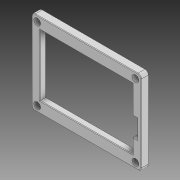
# Autodesk Inventor part: MainLid
Saved by Autodesk Inventor 2020 (Build 240168000, 168)
## iProperties
Created: 2021-01-12
Part Number: MainLid
Material: Generic
Document SubType Name: Modeling
Designer: DDeGo
Density: 1 g/cm^3
Appearance: Default
Author: DDeGo
Autodesk Inventor part; units mm, degrees
ref_plane "YZ Plane" through (0, 0, 0) normal (1, 0, 0) x (0, 1, 0)
ref_plane "XZ Plane" through (0, 0, 0) normal (0, 1, 0) x (-1, 0, 0)
ref_plane "XY Plane" through (0, 0, 0) normal (0, 0, 1) x (1, 0, 0)
sketch "Sketch1" plane through (0, 0, 0) normal (0, 0, 1) x (1, 0, 0)
  line L0 (46, -37.5) -> (-46, -37.5)
  line L1 (-49, -34.5) -> (-49, 34.5)
  line L2 (-46, 37.5) -> (46, 37.5)
  line L3 (49, 34.5) -> (49, -34.5)
  line L4 (49, -37.5) -> (-49, 37.5) construction
  line L5 (-49, -37.5) -> (49, 37.5) construction
  line L6 (44, -32.5) -> (-44, -32.5) construction
  line L7 (-44, -32.5) -> (-44, 32.5) construction
  line L8 (-44, 32.5) -> (44, 32.5) construction
  line L9 (44, 32.5) -> (44, -32.5) construction
  line L10 (44, -32.5) -> (-44, 32.5) construction
  line L11 (-44, -32.5) -> (44, 32.5) construction
  arc A0 (-46, 37.5) -> (-49, 34.5) centre (-46, 34.5) ccw
  arc A1 (49, 34.5) -> (46, 37.5) centre (46, 34.5) ccw
  arc A2 (46, -37.5) -> (49, -34.5) centre (46, -34.5) ccw
  circle A3 centre (-44, 32.5) radius 1.65
  circle A4 centre (-44, -32.5) radius 1.65
  circle A5 centre (44, -32.5) radius 1.65
  circle A6 centre (44, 32.5) radius 1.65
  arc A7 (-49, -34.5) -> (-46, -37.5) centre (-46, -34.5) ccw
  point P0 (0, 0)
  dimension "d0" = 75
  dimension "d1" = 98
  dimension "d2" = 3
  dimension "d3" = 88
  dimension "d4" = 65
  dimension "d5" = 3.3
  dimension "d6" = 3
  constraints: 24 end point, 8 centre point, 8 point on circle, 8 point on line, 8 tangent, 5 equal radius, 4 coincident, 4 midpoint, 4 parallel, 2 horizontal, 2 perpendicular
  measures "d0" distance of L5.start L4.end
  measures "d1" distance of L4.end L5.end
  measures "d2" radius of A0
  measures "d3" distance of L7.end L8.end
  measures "d4" distance of L6.end L7.end
  measures "d5" diameter of A3
  measures "d6" radius of A7
extrude "Extrusion1" add sketch "Sketch1" along normal blind 5
sketch "Sketch2" plane through (0, 0, 5) normal (0, 0, 1) x (1, 0, 0)
  line L0 (-41.5, -27.5) -> (41.5, -27.5)
  line L1 (41.5, 27.5) -> (-41.5, 27.5)
  line L2 (-41.5, 27.5) -> (-41.5, -27.5)
  line L3 (-41.5, -27.5) -> (41.5, 27.5) construction
  line L4 (41.5, -27.5) -> (-41.5, 27.5) construction
  line L5 (41.5, 2.5) -> (45.5, 2.5)
  line L6 (45.5, 2.5) -> (45.5, -14.5)
  line L7 (45.5, -14.5) -> (41.5, -14.5)
  line L8 (41.5, -27.5) -> (41.5, -14.5)
  line L9 (41.5, 2.5) -> (41.5, 27.5)
  point P0 (0, 0)
  dimension "d9" = 55
  dimension "d10" = 83
  dimension "d11" = 13
  dimension "d12" = 4
  dimension "d13" = 30
  constraints: 20 end point, 4 parallel, 3 perpendicular, 2 horizontal, 2 midpoint, 1 collinear
  measures "d9" distance of L0.end L1.start
  measures "d10" distance of L1.start L1.end
  measures "d11" distance between parallel lines of L0 L7
  measures "d12" distance of L6.end L7.end
  measures "d13" distance between parallel lines of L0 L5
extrude "Extrusion2" cut sketch "Sketch2" against normal through all
sketch "Sketch3" plane through (0, 0, 0) normal (0, 0, -1) x (-1, 0, 0)
  line L0 (41.5, -27.5) -> (-41.5, -27.5) projected
  line L1 (-41.5, -27.5) -> (-41.5, -14.5) projected
  line L2 (-41.5, -14.5) -> (-45.5, -14.5) construction
  line L3 (-45.5, -14.5) -> (-45.5, 2.5) construction
  line L4 (-45.5, 2.5) -> (-41.5, 2.5) construction
  line L5 (-41.5, 2.5) -> (-41.5, 27.5) projected
  line L6 (-41.5, 27.5) -> (41.5, 27.5) projected
  line L7 (41.5, 27.5) -> (41.5, -27.5) projected
  arc A0 (-49, -34.5) -> (-46, -37.5) centre (-46, -34.5) ccw projected
  line L8 (46, -37.5) -> (-46, -37.5) projected
  arc A1 (46, -37.5) -> (49, -34.5) centre (46, -34.5) ccw projected
  line L9 (49, 34.5) -> (49, -34.5) projected
  arc A2 (49, 34.5) -> (46, 37.5) centre (46, 34.5) ccw projected
  line L10 (-46, 37.5) -> (46, 37.5) projected
  arc A3 (-46, 37.5) -> (-49, 34.5) centre (-46, 34.5) ccw projected
  line L11 (-49, -34.5) -> (-49, 34.5) projected
  circle A4 centre (-44, 32.5) radius 1.65 projected
  circle A5 centre (-44, -32.5) radius 1.65 projected
  circle A6 centre (44, -32.5) radius 1.65 projected
  circle A7 centre (44, 32.5) radius 1.65 projected
  line L12 (43.5, -29.5) -> (-43.5, -29.5)
  line L13 (-43.5, -29.5) -> (-43.5, 29.5)
  line L14 (-43.5, 29.5) -> (43.5, 29.5)
  line L15 (43.5, 29.5) -> (43.5, -29.5)
  line L16 (43.5, -29.5) -> (-43.5, 29.5) construction
  line L17 (-43.5, -29.5) -> (43.5, 29.5) construction
  point P0 (0, 0)
  dimension "d16" = 2
  dimension "d17" = 2
  constraints: 12 end point, 2 midpoint, 2 parallel, 1 horizontal, 1 perpendicular
  measures "d16" distance between parallel lines of L6 L14
  measures "d17" distance between parallel lines of L13 L5
extrude "Extrusion3" add sketch "Sketch3" along normal blind 1.5
sketch "Sketch4" plane through (0, 0, -1.5) normal (0, 0, -1) x (-1, 0, 0)
  line L0 (30, -33) -> (-30, -33) construction
  line L1 (-30, -33) -> (-30, 33) construction
  line L2 (-30, 33) -> (30, 33) construction
  line L3 (30, 33) -> (30, -33) construction
  line L4 (30, -33) -> (-30, 33) construction
  line L5 (-30, -33) -> (30, 33) construction
  circle A0 centre (-30, 33) radius 1.2
  circle A1 centre (30, 33) radius 1.2
  circle A2 centre (-30, -33) radius 1.2
  circle A3 centre (30, -33) radius 1.2
  line L6 (46, 37.5) -> (-46, 37.5) projected
  circle A4 centre (0, 33) radius 1.2
  circle A5 centre (0, -33) radius 1.2
  point P0 (0, 0)
  dimension "d20" = 2.4
  dimension "d21" = 4.5
  dimension "d22" = 60
  constraints: 12 end point, 6 centre point, 5 equal radius, 4 coincident, 4 midpoint, 2 parallel, 1 horizontal, 1 perpendicular
  measures "d20" diameter of A0
  measures "d21" distance between parallel lines of L6 L2
  measures "d22" distance of L1.end L2.end
extrude "Extrusion4" cut sketch "Sketch4" against normal blind 5
sketch "Sketch5" plane through (0, 0, 0) normal (0, 0, 1) x (1, 0, 0)
  line L0 (45.5, 2.5) -> (43.5, 2.5) projected
  line L1 (43.5, -14.5) -> (43.5, 2.5) projected
  line L2 (43.5, -14.5) -> (45.5, -14.5) projected
  line L3 (45.5, -14.5) -> (45.5, 2.5) projected
  point P0 (0, 0)
extrude "Extrusion5" cut sketch "Sketch5" against normal blind 5
sketch "Sketch6" plane through (0, 0, 5) normal (0, 0, 1) x (1, 0, 0)
  circle A0 centre (-44, 32.5) radius 1.65 projected
  circle A1 centre (-44, 32.5) radius 3
  circle A2 centre (44, 32.5) radius 1.65 projected
  circle A3 centre (44, 32.5) radius 3
  circle A4 centre (44, -32.5) radius 1.65 projected
  circle A5 centre (44, -32.5) radius 3
  circle A6 centre (-44, -32.5) radius 1.65 projected
  circle A7 centre (-44, -32.5) radius 3
  point P0 (0, 0)
  dimension "d27" = 6
  constraints: 4 centre point, 4 coincident, 3 equal radius
  measures "d27" diameter of A1
extrude "Extrusion6" cut sketch "Sketch6" against normal blind 3 contours A0 | A1 | A2 | A3 | A4 | A5 | A6 | A7
chamfer "Chamfer1" distance 0.5 angle 45 15 edges at (49, 0, 5) (48.1213, 36.6213, 5) (0, 37.5, 5) (-48.1213, 36.6213, 5) (-49, 0, 5) (-48.1213, -36.6213, 5) (0, -37.5, 5) (48.1213, -36.6213, 5) (45.5, -6, 5) (43.5, 2.5, 5) (41.5, 15, 5) (0, 27.5, 5) (0, -27.5, 5) (41.5, -21, 5) (-41.5, 0, 5)
body "Solid1"
